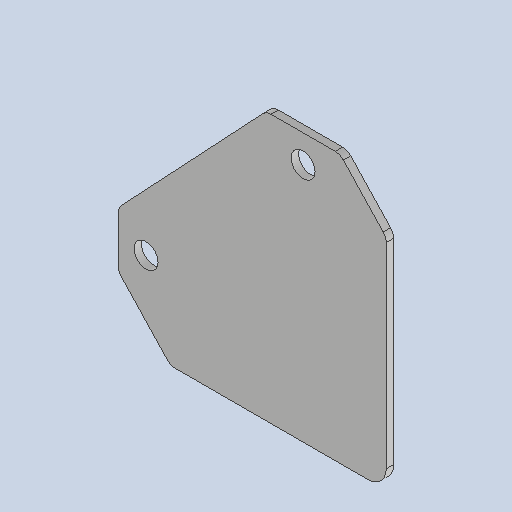
# Autodesk Inventor part: MSC 902 FLANGE FRAME HEEL
Saved by Autodesk Inventor 2025 (Build 290162010, 162A)
## iProperties
Created: 2024-07-01
Part Number: MSC 902 FLANGE FRAME HEEL
Material: Stainless Steel
Document SubType Name: Sheet Metal
Designer: pokla
Density: 8 g/cm^3
Sheet Metal Rule: AISI304 4mm Die 32
Appearance: Default
Stock Number: МОО 902 опора рамы
Mass: 530.491 g
Surface Area: 354.574 cm^2
Volume: 66.3114 cm^3
Flat Pattern Width: 14.2575 cm
Flat Pattern Length: 16.8189 cm
Flat Pattern Area: 239.796 cm^2
Sheet Metal Width: 142,575 mm
Sheet Metal Length: 168,189 mm
Sheet Metal Area: 23979,637 mm^2
Author: pokla
Autodesk Inventor part; units mm, degrees
ref_plane "YZ Plane" through (0, 0, 0) normal (1, 0, 0) x (0, 1, 0)
ref_plane "XZ Plane" through (0, 0, 0) normal (0, 1, 0) x (-1, 0, 0)
ref_plane "XY Plane" through (0, 0, 0) normal (0, 0, 1) x (1, 0, 0)
sketch "Sketch1" plane through (0, 0, 0) normal (0, 1, 0) x (-1, 0, 0)
  line L0 (40, 40) -> (-40, 40) construction
  line L1 (-40, 40) -> (-40, -40) construction
  line L2 (-40, -40) -> (40, -40) construction
  line L3 (40, -40) -> (40, 40) construction
  line L4 (-40, 40) -> (40, -40) construction
  line L5 (100, -45) -> (-100, -45)
  line L6 (-100, -45) -> (-100, 100)
  line L7 (-100, 100) -> (100, 100)
  line L8 (100, 100) -> (100, -45)
  circle A0 centre (85, 0) radius 6.5
  circle A1 centre (0, 85) radius 6.5
  circle A2 centre (-85, 0) radius 6.5
  line L9 (0, 40) -> (0, -40) construction
  line L10 (100, 15) -> (20, 100)
  line L11 (-20, 100) -> (-100, 15)
  line L12 (100, -15) -> (71.7647, -45)
  line L13 (-100, -15) -> (-71.7647, -45)
  line L14 (0, 0) -> (-40, 0) construction
  line L15 (-45, -45) -> (-45, 73.4375)
  point P0 (0, 0)
  point P1 (0, 0)
  dimension "d2" = 80
  dimension "d3" = 80
  dimension "d17" = 5
  dimension "d18" = 13
  dimension "d19" = 45
  dimension "d20" = 45
  dimension "d21" = 40
  dimension "d22" = 15
  dimension "d23" = 15
  dimension "d24" = 30
  dimension "d26" = 5
  measures "d2" distance of L2.end L1.end
  measures "d3" distance of L1.end L0.end
  measures "d17" distance between parallel lines of L5 L2
  measures "d18" diameter of A1
  measures "d19" distance from line of A1.centre L0
  measures "d20" distance from line of L1 A2.centre
  measures "d21" distance of L11.start L10.end
  measures "d22" distance from line of L7 A1.centre
  measures "d23" distance from line of L6 A2.centre
  measures "d24" distance of L13.start L11.end
  measures "d26" distance between parallel lines of L1 L15
extrude "Plate1" add sketch "Sketch1" along normal blind 4 contours L5 L15 L11 L7 L10 L8 L12
fillet "Corner Round2" radius 6 6 edges at (-20, 2, 100) (20, 2, 100) (-100, 2, 15) (-100, 2, -15) (-71.7647, 2, -45) (45, 2, 73.4375)
fillet "Corner Round4" radius 10 1 edges at (45, 2, -45)
equation "\"d20\" = d19"
equation "\"d23\" = d22"
equation "\"d26\" = d17"
equation "\"d6\" = Thickness"
equation "\"BendReliefWidth\" = Thickness"
equation "\"BendReliefDepth\" = 0.5 * Thickness"
equation "\"CornerReliefSize\" = 4 * Thickness"
equation "\"MinimumRemnant\" = 2 * Thickness"
equation "\"TransitionRadius\" = BendRadius"
equation "\"JacobiRadiusSize\" = BendRadius"
equation "\"GapSize\" = Thickness"
equation "\"Thickness\" = 4"
equation "\"BendRadius\" = 6"
body "Solid1"
